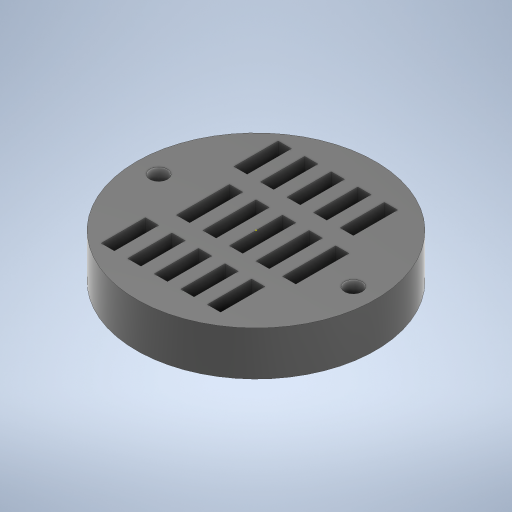
# Autodesk Inventor part: Acrylic_Seperator
Saved by Autodesk Inventor 2023 (Build 270158000, 158)
## iProperties
Created: 2022-09-10
Part Number: Acrylic_Seperator
Material: Generic
Document SubType Name: Modeling
Designer: Desmond
Density: 1 g/cm^3
Appearance: Default
Author: Desmond
Autodesk Inventor part; units mm, degrees
ref_plane "YZ Plane" through (0, 0, 0) normal (1, 0, 0) x (0, 1, 0)
ref_plane "XZ Plane" through (0, 0, 0) normal (0, 1, 0) x (-1, 0, 0)
ref_plane "XY Plane" through (0, 0, 0) normal (0, 0, 1) x (1, 0, 0)
sketch "Sketch1" plane through (0, 0, 0) normal (0, 1, 0) x (-1, 0, 0)
  circle A0 centre (0, 0) radius 13.5
  dimension "d0" = 27
  constraints: 1 centre point, 1 coincident
  measures "d0" diameter of A0
extrude "Extrusion1" add sketch "Sketch1" along normal blind 5
sketch "Sketch2" plane through (0, 5, 0) normal (0, 1, 0) x (1, 0, 0)
  line L0 (7.5, -10) -> (7.5, 10)
  line L1 (7.5, 10) -> (-7.5, 10)
  circle A0 centre (0, 0) radius 13.5 projected
  line L2 (-7.5, -10) -> (-6, -10)
  line L3 (-6, -10) -> (-6, -5)
  line L4 (-6, -5) -> (-7.5, -5)
  line L5 (-7.5, -5) -> (-7.5, -10)
  line L6 (-7.5, 5) -> (-6, 5)
  line L7 (-6, 5) -> (-6, 10)
  line L8 (-6, 10) -> (-7.5, 10)
  line L9 (-7.5, 10) -> (-7.5, 5)
  line L10 (-6, -3) -> (-4.5, -3)
  line L11 (-4.5, -3) -> (-4.5, 3)
  line L12 (-4.5, 3) -> (-6, 3)
  line L13 (-6, 3) -> (-6, -3)
  line L14 (-4.5, -10) -> (-3, -10)
  line L15 (-3, -10) -> (-3, -5)
  line L16 (-3, -5) -> (-4.5, -5)
  line L17 (-4.5, -5) -> (-4.5, -10)
  line L18 (-4.5, 5) -> (-3, 5)
  line L19 (-4.5, 10) -> (-4.5, 5)
  line L20 (-3, 5) -> (-3, 10)
  line L21 (-3, 10) -> (-4.5, 10)
  line L22 (-3, -3) -> (-1.5, -3)
  line L23 (-1.5, -3) -> (-1.5, 3)
  line L24 (-1.5, 3) -> (-3, 3)
  line L25 (-3, 3) -> (-3, -3)
  line L26 (-1.5, -10) -> (0, -10)
  line L27 (0, -10) -> (0, -5)
  line L28 (0, -5) -> (-1.5, -5)
  line L29 (-1.5, -5) -> (-1.5, -10)
  line L30 (-1.5, 5) -> (0, 5)
  line L31 (-1.5, 10) -> (-1.5, 5)
  line L32 (0, 5) -> (0, 10)
  line L33 (0, 10) -> (-1.5, 10)
  line L34 (0, -3) -> (1.5, -3)
  line L35 (1.5, -3) -> (1.5, 3)
  line L36 (1.5, 3) -> (0, 3)
  line L37 (0, 3) -> (0, -3)
  line L38 (1.5, -10) -> (3, -10)
  line L39 (3, -10) -> (3, -5)
  line L40 (3, -5) -> (1.5, -5)
  line L41 (1.5, -5) -> (1.5, -10)
  line L42 (1.5, 5) -> (3, 5)
  line L43 (1.5, 10) -> (1.5, 5)
  line L44 (3, 5) -> (3, 10)
  line L45 (3, 10) -> (1.5, 10)
  line L46 (3, -3) -> (4.5, -3)
  line L47 (4.5, -3) -> (4.5, 3)
  line L48 (4.5, 3) -> (3, 3)
  line L49 (3, 3) -> (3, -3)
  line L50 (4.5, -10) -> (6, -10)
  line L51 (6, -10) -> (6, -5)
  line L52 (6, -5) -> (4.5, -5)
  line L53 (4.5, -5) -> (4.5, -10)
  line L54 (4.5, 5) -> (6, 5)
  line L55 (4.5, 10) -> (4.5, 5)
  line L56 (6, 5) -> (6, 10)
  line L57 (6, 10) -> (4.5, 10)
  line L58 (6, -3) -> (7.5, -3)
  line L59 (7.5, -3) -> (7.5, 3)
  line L60 (7.5, 3) -> (6, 3)
  line L61 (6, 3) -> (6, -3)
  line L62 (-7.5, -10) -> (-7.5, 10)
  line L63 (7.5, -10) -> (-7.5, -10)
  point P0 (-4.5, 5)
  point P1 (-1.5, 5)
  point P2 (1.5, -5)
  point P3 (1.5, 5)
  point P4 (4.5, -5)
  point P5 (4.5, 5)
  point P6 (7.5, -5)
  point P7 (7.5, 5)
  dimension "d4" = 20
  dimension "d5" = 15
  dimension "d8" = 1.5
  dimension "d9" = 5
  dimension "d10" = 1.5
  dimension "d11" = 5
  dimension "d14" = 1.5
  dimension "d16" = 2
  dimension "d25" = 1.5
  dimension "d26" = 5
  dimension "d27" = 1.5
  dimension "d29" = 1.5
  dimension "d31" = 1.5
  dimension "d32" = 5
  dimension "d33" = 1.5
  dimension "d35" = 1.5
  dimension "d37" = 1.5
  dimension "d38" = 5
  dimension "d39" = 1.5
  dimension "d41" = 1.5
  dimension "d43" = 1.5
  dimension "d44" = 5
  dimension "d45" = 1.5
  dimension "d47" = 1.5
  dimension "d49" = 20
  dimension "d50" = 15
  constraints: 128 end point, 30 parallel, 15 horizontal, 15 perpendicular
  measures "d4" distance of L0.start L0.end
  measures "d5" distance of L0.end L1.end
  measures "d8" distance of L3.end L4.end
  measures "d9" distance of L2.end L3.end
  measures "d10" distance of L7.end L9.start
  measures "d11" distance of L6.end L7.end
  measures "d14" distance of L11.end L12.end
  measures "d16" distance between parallel lines of L4 L10
  measures "d25" distance of L15.end L17.start
  measures "d26" distance of L14.end L15.end
  measures "d27" distance of L20.end L19.start
  measures "d29" distance of L23.end L25.start
  measures "d31" distance of L27.end L29.start
  measures "d32" distance of L26.end L27.end
  measures "d33" distance of L32.end L31.start
  measures "d35" distance of L35.end L37.start
  measures "d37" distance of L39.end L41.start
  measures "d38" distance of L38.end L39.end
  measures "d39" distance of L44.end L43.start
  measures "d41" distance of L47.end L49.start
  measures "d43" distance of L51.end L53.start
  measures "d44" distance of L50.end L51.end
  measures "d45" distance of L56.end L55.start
  measures "d47" distance of L59.end L61.start
  measures "d49" distance of L62.start L62.end
  measures "d50" distance of L63.start L63.end
extrude "Extrusion2" cut sketch "Sketch2" against normal blind 5 contours L58 L61 L60 L0 | L50 L53 L52 L51 | L38 L41 L40 L39 | L56 L54 L55 L1 | L26 L29 L28 L27 | L44 L42 L43 L1 | L14 L17 L16 L15 | L32 L30 L31 L1 | L2 L5 L4 L3 | L20 L18 L19 L1 | L7 L6 L9 L1 | L13 L12 L11 L10 | L25 L24 L23 L22 | L37 L36 L35 L34 | L49 L48 L47 L46
sketch "Sketch3" plane through (0, 5, 0) normal (0, 1, 0) x (1, 0, 0)
  point P0 (0, 0)
sketch "Sketch4" plane through (0, 5, 0) normal (0, 1, 0) x (1, 0, 0)
  point P0 (0, 0)
sketch "Sketch5" plane through (0, 5, 0) normal (0, 1, 0) x (1, 0, 0)
  point P0 (0, 0)
sketch "Sketch6" plane through (0, 5, 0) normal (0, 1, 0) x (1, 0, 0)
  circle A0 centre (-11, 0) radius 1
  circle A1 centre (0, 0) radius 13.5 projected
  circle A2 centre (11, 0) radius 1
  line L0 (0, -3) -> (0, 3) projected
  dimension "d53" = 2
  dimension "d54" = 11
  dimension "d55" = 2
  dimension "d56" = 11
  constraints: 2 centre point
  measures "d53" diameter of A0
  measures "d54" distance of A1.centre A0.centre
  measures "d55" diameter of A2
  measures "d56" distance from line of L0 A2.centre
extrude "Extrusion3" cut sketch "Sketch6" against normal blind 5 contours A0 | A2
body "Solid1"
